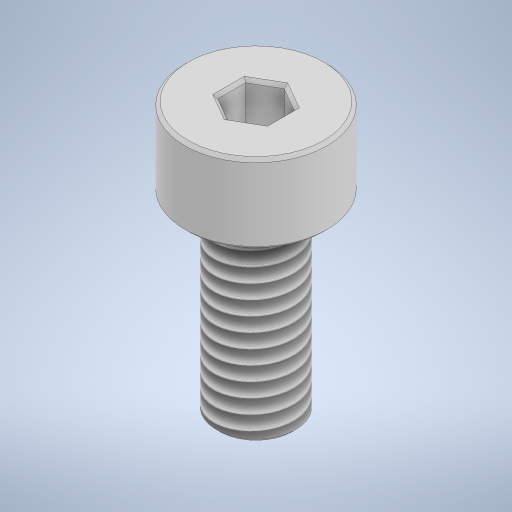
# Autodesk Inventor part: M2.5 X 6
Saved by Autodesk Inventor 2023 (Build 270158000, 158)
## iProperties
Created: 2023-04-10
Part Number: M2.5 X 6
Material: Generic
Document SubType Name: Modeling
Designer: Louis
Density: 1 g/cm^3
Appearance: Default
Author: Louis
Autodesk Inventor part; units mm, degrees
ref_plane "YZ Plane" through (0, 0, 0) normal (1, 0, 0) x (0, 1, 0)
ref_plane "XZ Plane" through (0, 0, 0) normal (0, 1, 0) x (-1, 0, 0)
ref_plane "XY Plane" through (0, 0, 0) normal (0, 0, 1) x (1, 0, 0)
sketch "Sketch1" plane through (0, 0, 0) normal (0, 0, 1) x (1, 0, 0)
  line L0 (0, 8.5) -> (2.25, 8.5)
  line L1 (2.25, 8.5) -> (2.25, 6)
  line L2 (2.25, 6) -> (1.25, 6)
  line L3 (1.25, 6) -> (1.25, 0)
  line L4 (1.25, 0) -> (0, 0)
  line L5 (0, 0) -> (0, 8.5)
  dimension "d0" = 2.25
  dimension "d1" = 2.5
  dimension "d2" = 6
  dimension "d3" = 1.25
  constraints: 12 end point, 5 perpendicular, 1 horizontal
  measures "d0" distance of L0.start L0.end
  measures "d1" distance of L0.end L1.end
  measures "d2" distance of L2.end L3.end
  measures "d3" distance of L3.end L4.end
revolve "Revolution1" add sketch "Sketch1" angle 360 about axis through (0, 0, 0) along (0, 1, 0)
thread "Thread1" size "M2.5x0.45" class "6g" standard "ANSI Metric M Profile" full length
sketch "Sketch3" plane through (0, 8.5, 0) normal (0, 1, 0) x (1, 0, 0)
  line L0 (0.77, -0.4446) -> (0, -0.8891)
  line L1 (0, -0.8891) -> (-0.77, -0.4446)
  line L2 (-0.77, -0.4446) -> (-0.77, 0.4446)
  line L3 (-0.77, 0.4446) -> (0, 0.8891)
  line L4 (0, 0.8891) -> (0.77, 0.4446)
  line L5 (0.77, 0.4446) -> (0.77, -0.4446)
  point P0 (0, 0)
  point P1 (0, 0)
  dimension "d13" = 1.54
  constraints: 12 end point, 1 coincident, 13 other
  measures "d13" distance between parallel lines of L5 L2
extrude "Extrusion2" cut sketch "Sketch3" against normal blind 1.5
chamfer "Chamfer2" distance 0.1 angle 45 16 edges at (0.385, 8.5, 0.6668) (0.77, 8.5, 0) (0.77, 7, 0) (0.385, 8.5, -0.6668) (0.385, 7, -0.6668) (-0.385, 8.5, -0.6668) (-0.385, 7, -0.6668) (-0.77, 7, 0) (-0.77, 8.5, 0) (-0.385, 7, 0.6668) (-0.385, 8.5, 0.6668) (0.385, 7, 0.6668) (-2.25, 8.5, 0) (-2.25, 6, 0) (-1.25, 6, 0) (-1.25, 0, 0)
body "Solid1"
